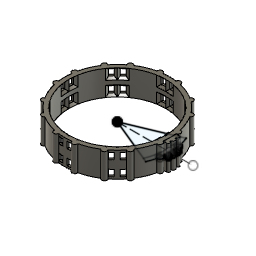
hard foot track v2 (Autodesk Fusion 360 design; units mm, degrees)
Autodesk Fusion 360 part; units mm, degrees
note: some values were not read from the file. Set by a fixed rule: which sketch regions a step uses.
sketch "layout" plane through (0, 0, 0) normal (0, 1, 0) x (1, 0, 0)
  line L0 (0, 0) -> (36.0109, 0) construction
  line L1 (25, -3) -> (26.5, -3)
  line L2 (26.5, -3) -> (26.5, 3)
  line L3 (26.5, 3) -> (25, 3)
  line L4 (25, 3) -> (25, -3)
  line L5 (25, -3) -> (26.5, 3) construction
  line L6 (26.5, -3) -> (25, 3) construction
  circle A0 centre (26.5, 0) radius 1
  circle A1 centre (26.5, 2.25) radius 0.75
  circle A2 centre (26.5, -2.25) radius 0.75
  line L7 (0, 0) -> (23.097, 9.5671)
  line L8 (0, 0) -> (25, 0) construction
  line L9 (0, 0) -> (23.097, -9.5671)
  arc A3 (23.097, -9.5671) -> (23.097, 9.5671) centre (0, 0) ccw
  arc A4 (21.2492, -8.8017) -> (21.2492, 8.8017) centre (0, 0) ccw
  circle A5 centre (24.6191, 4.3472) radius 1.25
  circle A6 centre (24.6191, -4.3472) radius 1.25
  point P0 (25.75, 0)
  dimension "d1" = 50
  dimension "d2" = 46
  dimension "d5" = 1.5
  dimension "d6" = 6
  dimension "d7" = 2
  dimension "d8" = 1.5
  dimension "d9" = 1.5
  dimension "d17" = 22.5
  dimension "d23" = 2.5
  dimension "d24" = 1.4
  constraint coincident L0.start L7.start
  constraint horizontal L0
  constraint horizontal L1
  constraint perpendicular L1 L2
  constraint parallel L1 L3
  constraint parallel L2 L4
  constraint coincident L5 P0
  constraint coincident L6 P0
  constraint coincident L0 P0
  constraint midpoint L2 A0.centre
  constraint coincident L2 A1.centre
  constraint coincident L2 A2.centre
  constraint tangent L3 A1
  constraint tangent L1 A2
  constraint tangent L4 A3
  constraint horizontal L8
  constraint symmetric L0.start L8 L7.start
  constraint symmetric L7.end L8 L9.end
  constraint coincident L7 A4.end
  constraint coincident L9 A4.start
  constraint coincident A3 A5.centre
  constraint symmetric L0 A5 A6
  measures "d1" diameter of A3
  measures "d2" diameter of A4
  measures "d5" distance of L2.end L3.end
  measures "d6" distance of L1.end L2.end
  measures "d7" diameter of A0
  measures "d8" diameter of A1
  measures "d9" diameter of A2
  measures "d17" angle of L7 L8
  measures "d23" diameter of A5
  measures "d24" distance of L3.end A5.centre
extrude "Extrude1" add sketch "layout" along normal mid plane 12 contours L7 L9 A3 A4 A5 A6 | A3 A6 | A3 A6 | A3 A5 | A3 A5 makes body 1
extrude "Extrude2" add sketch "layout" along normal mid plane 12 separate body contours L1 L2 L3 L4 A0 A1 A2 | L2 A2 | L2 A2 | L2 A0 | L2 A0 | L2 A1 | L2 A1 makes body 2
sketch "pins" plane through (25, 0, 0) normal (-1, 0, 0) x (0, 0, 1)
  line L0 (3, -6) -> (3, 6)
  line L1 (3, 6) -> (-3, 6)
  line L2 (-3, 6) -> (-3, -6)
  line L3 (-3, -6) -> (3, -6)
  line L4 (0, 1.75) -> (0, 22.5)
  line L5 (-3, 0) -> (3, 0)
  line L6 (-3, 5) -> (-1, 5)
  line L7 (-1, 5) -> (-1, 2)
  line L8 (-1, 2) -> (-3, 2)
  line L9 (-3, 2) -> (-3, 5)
  line L10 (0, 0) -> (-9.5671, 0)
  line L11 (3, 5) -> (1, 5)
  line L12 (3, 2) -> (3, 5)
  line L13 (1, 5) -> (1, 2)
  line L14 (1, 2) -> (3, 2)
  line L15 (0, 0) -> (9.5671, 0)
  line L16 (-3, -5) -> (-1, -5)
  line L17 (-3, -2) -> (-3, -5)
  line L18 (-1, -5) -> (-1, -2)
  line L19 (-1, -2) -> (-3, -2)
  line L20 (1, -5) -> (1, -2)
  line L21 (3, -5) -> (1, -5)
  line L22 (3, -2) -> (3, -5)
  line L23 (1, -2) -> (3, -2)
  dimension "d20" = 2
  dimension "d21" = 3
  dimension "d22" = 2
  constraint horizontal L6
  constraint vertical L7
  constraint horizontal L8
  constraint vertical L9
  constraint coincident L2 L6.start
  constraint symmetric L4 L6.start L11.start
  constraint symmetric L4 L6.end L11.end
  constraint symmetric L4 L7.end L13.end
  constraint symmetric L4 L8.end L12.start
  constraint symmetric L6.start L15 L16.start
  constraint symmetric L6.end L15 L16.end
  constraint symmetric L7.end L15 L18.end
  constraint symmetric L8.end L15 L17.start
  constraint symmetric L11.start L15 L21.start
  constraint symmetric L11.end L15 L20.start
  constraint symmetric L12.start L15 L22.start
  constraint symmetric L13.end L15 L20.end
  measures "d20" distance of L6.start L6.end
  measures "d21" distance of L6.start L8.end
  measures "d22" distance of L8 L10
extrude "Extrude3" add sketch "pins" along normal blind 3.5 contours L0 L20 L21 L22 L23 | L2 L16 L17 L18 L19 | L0 L11 L12 L13 L14 | L2 L6 L7 L8 L9 bodies 2
combine "Combine1" operation cut target body 1 tool bodies 2 keep tools
chamfer "Chamfer1" distance 1 angle 45 16 edges at (22.8035, 3.5, -3) (22.8035, -3.5, 3) (22.8035, -3.5, -3) (22.8035, 3.5, 3) (22.9127, 5, -2.0019) (22.9783, 3.5, -1) (22.9127, 2, -2.0019) (22.9127, -2, -2.0019) (22.9783, -3.5, -1) (22.9127, -5, -2.0019) (22.9783, 3.5, 1) (22.9127, 5, 2.0019) (22.9127, 2, 2.0019) (22.9127, -2, 2.0019) (22.9783, -3.5, 1) (22.9127, -5, 2.0019) on bodies 1
pattern_circular "C-Pattern1" count 8 over 360 about axis through (0, 1.75, 0) along (0, 1, 0) of bodies 1 makes body 3 at (20.5527, -0.3334, -10.3241) makes body 4 at (7.2327, -0.3334, -21.8332) makes body 5 at (-10.3241, -0.3334, -20.5527) makes body 6 at (-21.8332, -0.3334, -7.2327) makes body 7 at (-20.5527, -0.3334, 10.3241) makes body 8 at (-7.2327, -0.3334, 21.8332) makes body 9 at (10.3241, -0.3334, 20.5527)
combine "Combine2" operation add target body 1 tool bodies 3 4 5 6 7 8 9
equation "d17 = ( 360 / 16 ) * 1 deg"
named bodies: "track foot", "track track"
